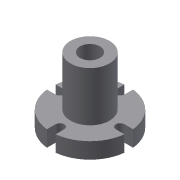
# Autodesk Inventor part: Nut
Saved by Autodesk Inventor 2014 (Build 180170000, 170)
## iProperties
Created: 2014-08-29
Part Number: Nut
Material: Generic
Document SubType Name: Modeling
Designer: Peele
Density: 1 g/cm^3
Appearance: Default
Author: Peele
Autodesk Inventor part; units mm, degrees
ref_plane "YZ Plane" through (0, 0, 0) normal (1, 0, 0) x (0, 1, 0)
ref_plane "XZ Plane" through (0, 0, 0) normal (0, 1, 0) x (-1, 0, 0)
ref_plane "XY Plane" through (0, 0, 0) normal (0, 0, 1) x (1, 0, 0)
sketch "Sketch1" plane through (0, 0, 0) normal (0, 0, 1) x (1, 0, 0)
  circle A0 centre (0, 0) radius 15.75
  circle A1 centre (0, 0) radius 4.05
  dimension "d0" = 31.5
  dimension "d1" = 8.1
  constraints: 2 centre point, 2 coincident
  measures "d0" diameter of A0
  measures "d1" diameter of A1
extrude "Extrusion1" add sketch "Sketch1" along normal blind 6.46
sketch "Sketch2" plane through (0, 0, 6.46) normal (0, 0, 1) x (1, 0, 0)
  circle A0 centre (0, 0) radius 4.05 projected
  circle A1 centre (0, 0) radius 15.75 projected
  circle A2 centre (0, 0) radius 7.9
  circle A3 centre (0, 0) radius 4.05
  dimension "d4" = 15.8
  constraints: 2 centre point, 2 coincident, 1 concentric
  measures "d4" diameter of A2
extrude "Extrusion2" add sketch "Sketch2" along normal blind 20 contours A2
sketch "Sketch3" plane through (0, 0, 0) normal (0, 0, -1) x (-1, 0, 0)
  circle A0 centre (0, 0) radius 4.05 projected
  circle A1 centre (0, 0) radius 15.75 projected
  line L0 (-1.75, 15.6525) -> (-1.75, 12.1525)
  line L1 (1.75, 12.1525) -> (1.75, 15.6525)
  arc A2 (-1.75, 12.1525) -> (1.75, 12.1525) centre (0, 12.1525) ccw
  arc A3 (1.75, 15.6525) -> (-1.75, 15.6525) centre (0, 0) ccw
  dimension "d7" = 3.5
  dimension "d8" = 3.5
  constraints: 6 point on circle, 4 end point, 2 centre point, 2 tangent, 1 concentric, 1 parallel, 1 vertical, 1 vertical alignment
  measures "d7" distance between parallel lines of L0 L1
  measures "d8" vertical distance of A2.centre L1.end
extrude "Extrusion3" cut sketch "Sketch3" against normal blind 20 contours L1 A2 L0 A1 picked at (0.1948, 13.3481)
pattern_circular "Circular Pattern1" count 4 over 360 about axis through (0, 0, 0) along (0, 0, 1) of "Extrusion3"
body "Solid1"
